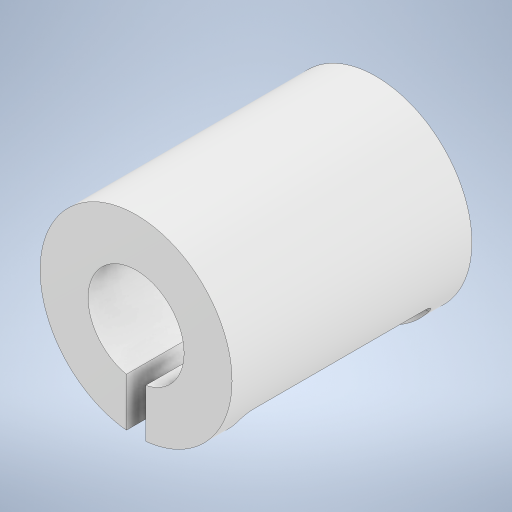
# Autodesk Inventor part: StoperKlein
Saved by Autodesk Inventor 2024.4 (Build 284460000, 460)
## iProperties
Created: 2026-01-10
Part Number: StoperKlein
Material: PVC, hart
Description: StoperKlein
Document SubType Name: Modeling
Designer: Philf
Mass: 55.5783 g
Surface Area: 124.769 cm^2
Volume: 43.0839 cm^3
Density: 1.29 g/cm^3
Appearance: Glatt - Weiß
Masse[kg]: 0,076 kg
Autodesk Inventor part; units mm, degrees
ref_plane "YZ Plane" through (0, 0, 0) normal (1, 0, 0) x (0, 1, 0)
ref_plane "XZ Plane" through (0, 0, 0) normal (0, 1, 0) x (-1, 0, 0)
sketch "Skizze1" plane through (0, 0, 0) normal (0, 1, 0) x (-1, 0, 0)
  circle A0 centre (0, 0) radius 10
  circle A1 centre (0, 0) radius 20
  dimension "d0" = 20
  dimension "d1" = 40
  constraints: 2 centre point, 2 coincident
  measures "d0" diameter of A0
  measures "d1" diameter of A1
extrude "Extrusion1" add sketch "Skizze1" along normal blind 50
sketch "Skizze2" plane through (0, 50, 0) normal (0, 1, 0) x (1, 0, 0)
  line L0 (0, 0) -> (2, 0)
  line L1 (2, 0) -> (2, 25)
  line L2 (2, 25) -> (0, 25)
  line L3 (0, 25) -> (0, 0)
  line L4 (0, 0) -> (-2, 0)
  line L5 (-2, 0) -> (-2, 25)
  line L6 (-2, 25) -> (0, 25)
  line L7 (0, 25) -> (0, 0)
  dimension "d4" = 2
  dimension "d5" = 25
  dimension "d6" = 2
  dimension "d7" = 25
  constraints: 16 end point, 4 parallel, 2 horizontal, 2 perpendicular
  measures "d4" distance of L2.end L1.end
  measures "d5" distance of L1.end L0.end
  measures "d6" distance of L5.end L6.end
  measures "d7" distance of L4.end L5.end
extrude "Extrusion2" cut sketch "Skizze2" against normal blind 50
ref_plane "Arbeitsebene1" through (20, 0, 0) normal (1, 0, 0) x (0, 0, -1)
sketch "Skizze5" plane through (20, 0, 0) normal (1, 0, 0) x (0, 0, -1)
  line L0 (0, 0) -> (10, 0)
  line L1 (-10, 0) -> (9.798, 0) projected
  line L2 (10, 0) -> (10, 5)
  line L3 (10, 7) -> (10, 43)
  line L4 (12, 45) -> (18, 45)
  line L5 (20, 43) -> (20, 7)
  line L6 (18, 5) -> (12, 5)
  arc A0 (18, 5) -> (20, 7) centre (18, 7) ccw
  arc A1 (10, 7) -> (12, 5) centre (12, 7) ccw
  arc A2 (12, 45) -> (10, 43) centre (12, 43) ccw
  arc A3 (20, 43) -> (18, 45) centre (18, 43) ccw
  point P0 (10, 45)
  point P1 (20, 45)
  dimension "d11" = 10
  dimension "d12" = 5
  dimension "d13" = 40
  dimension "d14" = 10
  dimension "d15" = 2
  constraints: 12 end point, 8 point on circle, 8 tangent, 7 point on line, 4 centre point, 4 perpendicular, 3 equal radius, 1 collinear
  measures "d11" distance of L0.start L0.end
  measures "d12" distance of L0.end L2.end
  measures "d13" distance of L2.end point (10, 45)
  measures "d14" distance of point (10, 45) point (20, 45)
  measures "d15" radius of A0
extrude "Extrusion3" cut sketch "Skizze5" against normal blind 10
sketch "Skizze6" plane through (20, 0, 0) normal (1, 0, 0) x (0, 0, -1)
  line L0 (17.3205, 5) -> (12, 5) projected
  line L1 (15, 5) -> (15, 15)
  line L2 (15, 15) -> (15, 35)
  circle A0 centre (15, 15) radius 2.5
  circle A1 centre (15, 35) radius 2.5
  point P0 (0, 0)
  point P1 (18, 5)
  dimension "d18" = 10
  dimension "d19" = 20
  dimension "d20" = 5
  dimension "d21" = 5
  constraints: 4 end point, 2 centre point, 2 coincident, 2 point on line, 1 vertical
  measures "d18" distance of L1.start L1.end
  measures "d19" distance of L1.end L2.end
  measures "d20" diameter of A0
  measures "d21" diameter of A1
extrude "Extrusion4" cut sketch "Skizze6" against normal through all
thread "Gewinde1" size "M5x0.8" class "6H" standard "ANSI Metric M Profile" full length
sketch "Skizze8" plane through (20, 0, 0) normal (1, 0, 0) x (0, 0, -1)
  circle A0 centre (15, 35) radius 2.5 projected
  circle A1 centre (15, 35) radius 2.6
  arc A2 (17.3205, 15.9302) -> (17.3205, 14.0698) centre (15, 15) ccw projected
  circle A3 centre (15, 15) radius 2.6
  point P0 (0, 0)
  point P1 (14.8661, 37.4964)
  point P2 (14.8661, 32.5036)
  dimension "d30" = 5.2
  dimension "d31" = 5.2
  constraints: 2 centre point, 2 coincident
  measures "d30" diameter of A1
  measures "d31" diameter of A3
extrude "Extrusion6" cut sketch "Skizze8" against normal blind 25 contours A0 | A1 | A3
thread "Gewinde2" size "M5x0.8" class "6H" standard "ANSI Metric M Profile" full length
thread "Gewinde3" size "M5x0.8" class "6H" standard "ANSI Metric M Profile" full length
equation "\"d0\" = durchmesser"
equation "\"durchmesser\" = 20"
